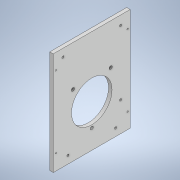
# Autodesk Inventor part: front plate
Saved by Autodesk Inventor 2020.3 (Build 243373000, 373)
## iProperties
Created: 2020-08-09
Part Number: front plate
Material: Generic
Document SubType Name: Modeling
Designer: joesp
Density: 1 g/cm^3
Appearance: Default
Author: joesp
Autodesk Inventor part; units mm, degrees
ref_plane "YZ Plane" through (0, 0, 0) normal (1, 0, 0) x (0, 1, 0)
ref_plane "XZ Plane" through (0, 0, 0) normal (0, 1, 0) x (-1, 0, 0)
ref_plane "XY Plane" through (0, 0, 0) normal (0, 0, 1) x (1, 0, 0)
sketch "Sketch1" plane through (0, 0, 0) normal (1, 0, 0) x (0, 1, 0)
  line L0 (0, 0) -> (147, 0)
  line L1 (147, 0) -> (147, 110)
  line L2 (147, 110) -> (0, 110)
  line L3 (0, 110) -> (0, 0)
  circle A0 centre (124.75, 106.25) radius 1
  circle A1 centre (124.75, 3.75) radius 1
  circle A2 centre (22.25, 3.75) radius 1
  circle A3 centre (22.25, 106.25) radius 1
  dimension "d0" = 102.5
  dimension "d1" = 102.5
  dimension "d2" = 2
  dimension "d3" = 110
  dimension "d4" = 147
  dimension "d5" = 22.25
  dimension "d6" = 22.25
  dimension "d7" = 3.75
  dimension "d8" = 3.75
  constraints: 8 end point, 4 centre point, 3 equal radius, 2 horizontal alignment, 2 parallel, 2 vertical alignment, 1 horizontal, 1 perpendicular
  measures "d0" distance of A1.centre A0.centre
  measures "d1" distance of A3.centre A0.centre
  measures "d2" diameter of A0
  measures "d3" distance of L0.end L1.end
  measures "d4" distance of L1.end L2.end
  measures "d5" distance from line of L1 A0.centre
  measures "d6" distance from line of L3 A3.centre
  measures "d7" distance from line of L2 A0.centre
  measures "d8" distance from line of L0 A1.centre
extrude "Extrusion1" add sketch "Sketch1" along normal blind 5
sketch "Sketch4" plane through (5, 0, 0) normal (1, 0, 0) x (0, 0, -1)
  circle A0 centre (-28, 88.9739) radius 2.25
  circle A1 centre (-82, 88.9739) radius 2.25
  circle A2 centre (-55, 27.6539) radius 2.25
  line L0 (-86.5, 89.2313) -> (-86.5, 45.9739)
  line L1 (-86.5, 45.9739) -> (-74.6331, 32.4396)
  arc A3 (-74.6331, 32.4396) -> (-35.3669, 32.4396) centre (-55, 49.6539) ccw
  line L2 (-35.3669, 32.4396) -> (-23.5, 45.9739)
  line L3 (-23.5, 45.9739) -> (-23.5, 89.2313)
  arc A4 (-80.5, 93.4739) -> (-86.5, 89.2313) centre (-82, 89.2313) ccw
  arc A5 (-23.5, 89.2313) -> (-29.5, 93.4739) centre (-28, 89.2313) ccw
  line L4 (-80.5, 93.4739) -> (-80.5, 97.4739)
  line L5 (-29.5, 93.4739) -> (-29.5, 97.4739)
  arc A6 (-29.5, 97.4739) -> (-80.5, 97.4739) centre (-55, 73.5) ccw
  line L6 (0, 0) -> (0, 147) projected
  line L7 (-110, 147) -> (-110, 0) projected
  line L8 (0, 147) -> (-110, 147) projected
  line L9 (-110, 0) -> (0, 0) projected
  circle A7 centre (-55, 60.6539) radius 29
  dimension "d38" = 54
  dimension "d39" = 63
  dimension "d40" = 51
  dimension "d43" = 6
  dimension "d44" = 6
  dimension "d45" = 61.32
  dimension "d46" = 43
  dimension "d47" = 18
  dimension "d48" = 4
  dimension "d49" = 4.5
  dimension "d50" = 4.5
  dimension "d51" = 4.5
  dimension "d52" = 4.5
  dimension "d55" = 35
  dimension "d56" = 22
  dimension "d57" = 23.5
  dimension "d58" = 23.5
  dimension "d59" = 4.5
  dimension "d60" = 4.5
  dimension "d61" = 73.5
  dimension "d62" = 73.5
  dimension "d63" = 58
  dimension "d64" = 33
  constraints: 12 end point, 8 centre point, 8 point on circle, 4 horizontal alignment, 4 tangent, 4 vertical, 3 equal length, 2 equal radius, 2 vertical alignment
  measures "d38" distance of A0.centre A1.centre
  measures "d39" distance between parallel lines of L3 L0
  measures "d40" distance between parallel lines of L5 L4
  measures "d43" distance between parallel lines of L0 L4
  measures "d44" distance between parallel lines of L3 L5
  measures "d45" vertical distance of A0.centre A2.centre
  measures "d46" vertical distance of L2.end A0.centre
  measures "d47" distance of L2.start L2.end
  measures "d48" distance of L5.start L5.end
  measures "d49" distance from line of L0 A1.centre
  measures "d50" vertical distance of L4.start A1.centre
  measures "d51" diameter of A1
  measures "d52" radius of A4
  measures "d55" radius of A6
  measures "d56" distance of A3.centre A2.centre
  measures "d57" distance between parallel lines of L6 L3
  measures "d58" distance between parallel lines of L7 L0
  measures "d59" vertical distance of L5.start A0.centre
  measures "d60" horizontal distance of L3.end A0.centre
  measures "d61" distance from line of L8 A6.centre
  measures "d62" distance from line of L9 A6.centre
  measures "d63" diameter of A7
  measures "d64" distance of A2.centre A7.centre
extrude "Extrusion3" cut sketch "Sketch4" against normal through all contours A0 | A1 | A2 | A7
sketch "Sketch5" plane through (5, 0, 0) normal (1, 0, 0) x (0, 0, -1)
  line L0 (-6, 0) -> (-6, 147)
  line L1 (-6, 147) -> (-104, 147)
  line L2 (-104, 147) -> (-104, 0)
  line L3 (-104, 0) -> (-6, 0)
  line L4 (-8, 2) -> (-8, 145)
  line L5 (-8, 145) -> (-102, 145)
  line L6 (-102, 145) -> (-102, 2)
  line L7 (-102, 2) -> (-8, 2)
  line L8 (-102, 137) -> (-102, 135)
  line L9 (-102, 135) -> (-99, 135)
  line L10 (-99, 135) -> (-99, 137)
  line L11 (-99, 137) -> (-102, 137)
  circle A0 centre (-96.1716, 136) radius 3
  line L12 (-8, 135) -> (-8, 133)
  line L13 (-8, 133) -> (-11, 133)
  line L14 (-11, 133) -> (-11, 135)
  line L15 (-11, 135) -> (-8, 135)
  circle A1 centre (-13.8284, 134) radius 3
  line L16 (-90, 2) -> (-90, 8)
  line L17 (-90, 8) -> (-88, 8)
  line L18 (-88, 8) -> (-88, 2)
  line L19 (-88, 2) -> (-90, 2)
  line L20 (-20, 2) -> (-20, 8)
  line L21 (-20, 8) -> (-22, 8)
  line L22 (-22, 8) -> (-22, 2)
  line L23 (-22, 2) -> (-20, 2)
  line L24 (-8, 41) -> (-8, 43)
  line L25 (-8, 43) -> (-11, 43)
  line L26 (-11, 43) -> (-11, 41)
  line L27 (-11, 41) -> (-8, 41)
  circle A2 centre (-89, 10.8284) radius 3
  circle A3 centre (-21, 10.8284) radius 3
  circle A4 centre (-13.8284, 42) radius 3
  line L28 (0, 0) -> (0, 147) projected
  line L29 (-110, 147) -> (-110, 0) projected
  line L30 (0, 147) -> (-110, 147) projected
  circle A5 centre (-96.1716, 136) radius 1.5
  circle A6 centre (-13.8284, 134) radius 1.5
  circle A7 centre (-21, 10.8284) radius 1.5
  circle A8 centre (-13.8284, 42) radius 1.5
  circle A9 centre (-89, 10.8284) radius 1.5
  dimension "d67" = 2
  dimension "d68" = 2
  dimension "d69" = 2
  dimension "d70" = 2
  dimension "d71" = 98
  dimension "d72" = 147
  dimension "d73" = 2
  dimension "d74" = 3
  dimension "d75" = 6
  dimension "d76" = 11
  dimension "d77" = 3
  dimension "d78" = 2
  dimension "d79" = 6
  dimension "d80" = 11
  dimension "d81" = 2
  dimension "d82" = 2
  dimension "d83" = 6
  dimension "d84" = 2
  dimension "d85" = 3
  dimension "d86" = 6
  dimension "d87" = 6
  dimension "d88" = 6
  dimension "d89" = 15
  dimension "d90" = 15
  dimension "d91" = 42
  dimension "d92" = 6
  dimension "d93" = 6
  dimension "d94" = 3
  constraints: 56 end point, 14 parallel, 10 centre point, 10 point on circle, 7 perpendicular, 6 coincident, 6 point on line, 4 equal radius, 3 horizontal, 3 vertical, 1 collinear
  measures "d67" distance between parallel lines of L1 L5
  measures "d68" distance between parallel lines of L2 L6
  measures "d69" distance between parallel lines of L0 L4
  measures "d70" distance between parallel lines of L7 L3
  measures "d71" distance between parallel lines of L0 L2
  measures "d72" distance between parallel lines of L1 L3
  measures "d73" distance between parallel lines of L11 L9
  measures "d74" distance of L11.start L11.end
  measures "d75" diameter of A0
  measures "d76" distance from line of L1 A0.centre
  measures "d77" distance of L15.start L15.end
  measures "d78" distance of L13.end L15.start
  measures "d79" diameter of A1
  measures "d80" distance from line of L5 A1.centre
  measures "d81" distance of L16.end L18.start
  measures "d82" distance of L21.start L21.end
  measures "d83" distance of L18.start L18.end
  measures "d84" distance of L26.start L26.end
  measures "d85" distance of L25.start L26.start
  measures "d86" diameter of A2
  measures "d87" diameter of A3
  measures "d88" diameter of A4
  measures "d89" distance from line of L2 A2.centre
  measures "d90" distance from line of L0 A3.centre
  measures "d91" distance from line of L3 A4.centre
  measures "d92" distance between parallel lines of L28 L0
  measures "d93" distance between parallel lines of L29 L2
  measures "d94" diameter of A5
extrude "Extrusion4" cut sketch "Sketch5" against normal through all contours A5 | A6 | A7 | A8 | A9
equation "\"d1\" = d0"
equation "\"d5\" = d6"
equation "\"d7\" = d8"
equation "\"d43\" = d44"
equation "\"d50\" = d49"
body "Solid1"
